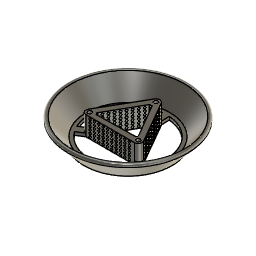
gaseta EMF medio v7 (Autodesk Fusion 360 design; units mm, degrees)
Autodesk Fusion 360 part; units mm, degrees
sketch "Boceto1" plane through (0, 0, 0) normal (0, 0, 1) x (1, 0, 0)
  circle A0 centre (0, 0) radius 55
  circle A1 centre (0, 35) radius 2
  circle A2 centre (-30.3109, -17.5) radius 2
  circle A3 centre (30.3109, -17.5) radius 2
  dimension "d1" = 110
  dimension "d2" = 4
  dimension "d4" = 360
  constraint coincident A0.centre origin
  measures "d1" diameter of A0
  measures "d2" diameter of A1
extrude "Extruir1" add sketch "Boceto1" along normal blind 4
sketch "Boceto2" plane through (0, 0, 0) normal (0, 1, 0) x (1, 0, 0)
  line L0 (55, 0) -> (78.3935, 0) construction
  line L1 (-55, 0) -> (55, 0) construction
  line L2 (55, 0) -> (74.2836, -22.9813)
  line L3 (70.7419, -25.9532) -> (51.4583, -2.9719)
  line L4 (51.4583, -2.9719) -> (55, 0)
  line L5 (-55, -4) -> (55, -4) construction
  arc A0 (70.7419, -25.9532) -> (74.2836, -22.9813) centre (72.5128, -24.4673) ccw
  dimension "d10" = 55
  dimension "d14" = 50
  dimension "d16" = 4
  constraint horizontal L0
  constraint parallel L2 L3
  measures "d10" distance of origin L0.start
  measures "d14" angle of L0 L2
  measures "d16" distance of L0 L5
revolve "Revolución1" add sketch "Boceto2" angle 360 about axis through (0, 0, 1.75) along (0, 0, 1)
sketch "Boceto3" plane through (0, 0, 4) normal (0, 0, 1) x (-1, 0, 0)
  circle A0 centre (0, 0) radius 52.321
  circle A1 centre (30.3109, 17.5) radius 2.5
  circle A2 centre (-30.3109, 17.5) radius 2.5
  line L0 (4.4101, -37.356) -> (34.7606, 15.2015)
  arc A3 (34.7534, 15.2057) -> (30.1462, 22.4973) centre (30.3109, 17.5) ccw
  line L1 (34.7606, 15.2015) -> (34.7534, 15.2057)
  line L2 (-0.0023, -25.0055) -> (21.6565, 12.5008)
  line L3 (21.6565, 12.5008) -> (-21.6543, 12.5047)
  arc A4 (34.7534, 15.2057) -> (30.1462, 22.4973) centre (30.3109, 17.5) ccw
  line L4 (30.1462, 22.4973) -> (-30.5452, 22.4945)
  arc A5 (-30.5452, 22.4945) -> (-34.6389, 15.0017) centre (-30.3098, 17.5012) ccw
  line L5 (-21.6543, 12.5047) -> (-0.0023, -25.0055)
  line L6 (-34.6389, 15.0017) -> (-4.2082, -37.7002)
  arc A6 (-4.2082, -37.7002) -> (4.4101, -37.356) centre (0, -35) ccw
  circle A7 centre (0, -35) radius 2.5
  dimension "d66" = 5
  dimension "d67" = 5
  dimension "d68" = 5
  constraint coincident L0 A6.end
  constraint coincident L6 A5.end
  constraint coincident L4.end A5.start
  constraint coincident A3.end A4.end
  constraint coincident L6.end A6.start
  constraint coincident A5.end L6.start
  constraint coincident L0.start A6.end
  constraint concentric A6 A7
  measures "d66" diameter of A1
  measures "d67" diameter of A2
  measures "d68" diameter of A7
extrude "Extruir2" add sketch "Boceto3" along normal blind 20 contours L0 A3 L1 A4 L4 A5 L6 A6 | L2 L3 L5
extrude "Extruir3" add sketch "Boceto3" along normal blind 20 contours L0 A3 L1 A4 L4 A5 L6 A6
extrude "Extruir4" cut sketch "Boceto3" against normal blind 30 contours A1 | A2 | A7
sketch "Boceto5" plane through (0, 0, 0) normal (0, 0, -1) x (1, 0, 0)
  circle A0 centre (-30.3109, 17.5) radius 2.5
  circle A1 centre (30.3109, 17.5) radius 2.5
  circle A2 centre (0, 0) radius 55
  line L0 (0.2076, -31) -> (27.1755, 15.0161)
  line L1 (27.1755, 15.0161) -> (-26.6179, 15.9631)
  line L2 (-26.6179, 15.9631) -> (0.2076, -31)
  arc A3 (-30.1462, 22.4973) -> (-34.7534, 15.2057) centre (-30.3109, 17.5) ccw
  line L3 (4.2082, -37.7002) -> (3.803, -47.8491)
  line L4 (-4.8254, -47.7568) -> (-4.4101, -37.356)
  line L5 (30.5452, 22.4945) -> (39.537, 27.218)
  line L6 (43.7713, 19.6995) -> (34.5563, 14.8588)
  line L7 (-34.7534, 15.2057) -> (-43.34, 20.6311)
  line L8 (-38.9459, 28.0573) -> (-30.1462, 22.4973)
  arc A4 (39.537, 27.218) -> (-38.9459, 28.0573) centre (0, 0) ccw
  arc A5 (-43.34, 20.6311) -> (-4.8254, -47.7568) centre (0, 0) ccw
  arc A6 (3.803, -47.8491) -> (43.7713, 19.6995) centre (0, 0) ccw
  line L9 (34.5563, 14.8588) -> (4.2082, -37.7002)
  line L10 (-4.4101, -37.356) -> (-34.7534, 15.2057)
  line L11 (-30.1462, 22.4973) -> (30.5452, 22.4945)
  circle A7 centre (0, -35) radius 2.5
  point P0 (0, -35)
  point P1 (30.3098, 17.5012)
  dimension "d31" = 4
  dimension "d32" = 4
  dimension "d33" = 4
  dimension "d34" = 96
  constraint coincident A3.end L7.start
  constraint coincident A3.start L8.end
  constraint coincident L5.end A5
  constraint concentric A4 A5
  constraint coincident L3.end A5
  constraint concentric A5 A6
  measures "d31" vertical distance of L0.start P0
  measures "d32" distance of L0.end P1
  measures "d33" distance of L1.end A0.centre
  measures "d34" diameter of A5
extrude "Extruir5" cut sketch "Boceto5" against normal blind 80 contours L0 L1 L2 | L3 L6 A6 L9 | L4 L7 A5 L10 | L5 L8 A4 L11
fillet "Empalme1" radius 2 3 edges at (27.1755, -15.0161, 12) (-26.6179, -15.9631, 12) (0.2076, 31, 12)
sketch "Boceto6" plane through (-19.4825, 11.2471, 0) normal (-0.866048, 0.49996, 0) x (-0.49996, -0.866048, 0)
  line L0 (30.5442, 24) -> (-30.1473, 24)
  line L1 (-30.1473, 24) -> (-30.1473, 4)
  line L2 (-30.1473, 4) -> (-30.1473, 0)
  line L3 (-30.1473, 0) -> (30.5442, 0)
  line L4 (30.5442, 0) -> (30.5442, 4)
  line L5 (30.5442, 4) -> (30.5442, 24)
  circle A0 centre (-25, 21.5) radius 1.35
  circle A1 centre (-19.4444, 21.5) radius 1.35
  circle A2 centre (-13.8889, 21.5) radius 1.35
  circle A3 centre (-8.3333, 21.5) radius 1.35
  circle A4 centre (-2.7778, 21.5) radius 1.35
  circle A5 centre (2.7778, 21.5) radius 1.35
  circle A6 centre (8.3333, 21.5) radius 1.35
  circle A7 centre (13.8889, 21.5) radius 1.35
  circle A8 centre (19.4444, 21.5) radius 1.35
  circle A9 centre (25, 21.5) radius 1.35
  circle A10 centre (-25, 17.7) radius 1.35
  circle A11 centre (-19.4444, 17.7) radius 1.35
  circle A12 centre (-13.8889, 17.7) radius 1.35
  circle A13 centre (-8.3333, 17.7) radius 1.35
  circle A14 centre (-2.7778, 17.7) radius 1.35
  circle A15 centre (2.7778, 17.7) radius 1.35
  circle A16 centre (8.3333, 17.7) radius 1.35
  circle A17 centre (13.8889, 17.7) radius 1.35
  circle A18 centre (19.4444, 17.7) radius 1.35
  circle A19 centre (25, 17.7) radius 1.35
  circle A20 centre (-25, 13.9) radius 1.35
  circle A21 centre (-19.4444, 13.9) radius 1.35
  circle A22 centre (-13.8889, 13.9) radius 1.35
  circle A23 centre (-8.3333, 13.9) radius 1.35
  circle A24 centre (-2.7778, 13.9) radius 1.35
  circle A25 centre (2.7778, 13.9) radius 1.35
  circle A26 centre (8.3333, 13.9) radius 1.35
  circle A27 centre (13.8889, 13.9) radius 1.35
  circle A28 centre (19.4444, 13.9) radius 1.35
  circle A29 centre (25, 13.9) radius 1.35
  circle A30 centre (-25, 10.1) radius 1.35
  circle A31 centre (-19.4444, 10.1) radius 1.35
  circle A32 centre (-13.8889, 10.1) radius 1.35
  circle A33 centre (-8.3333, 10.1) radius 1.35
  circle A34 centre (-2.7778, 10.1) radius 1.35
  circle A35 centre (2.7778, 10.1) radius 1.35
  circle A36 centre (8.3333, 10.1) radius 1.35
  circle A37 centre (13.8889, 10.1) radius 1.35
  circle A38 centre (19.4444, 10.1) radius 1.35
  circle A39 centre (25, 10.1) radius 1.35
  circle A40 centre (-25, 6.3) radius 1.35
  circle A41 centre (-19.4444, 6.3) radius 1.35
  circle A42 centre (-13.8889, 6.3) radius 1.35
  circle A43 centre (-8.3333, 6.3) radius 1.35
  circle A44 centre (-2.7778, 6.3) radius 1.35
  circle A45 centre (2.7778, 6.3) radius 1.35
  circle A46 centre (8.3333, 6.3) radius 1.35
  circle A47 centre (13.8889, 6.3) radius 1.35
  circle A48 centre (19.4444, 6.3) radius 1.35
  circle A49 centre (25, 6.3) radius 1.35
  circle A50 centre (-25, 2.5) radius 1.35
  circle A51 centre (-19.4444, 2.5) radius 1.35
  circle A52 centre (-13.8889, 2.5) radius 1.35
  circle A53 centre (-8.3333, 2.5) radius 1.35
  circle A54 centre (-2.7778, 2.5) radius 1.35
  circle A55 centre (2.7778, 2.5) radius 1.35
  circle A56 centre (8.3333, 2.5) radius 1.35
  circle A57 centre (13.8889, 2.5) radius 1.35
  circle A58 centre (19.4444, 2.5) radius 1.35
  circle A59 centre (25, 2.5) radius 1.35
  dimension "d39" = 2.7
  dimension "d42" = 50
  dimension "d43" = -19
  dimension "d44" = 21.5
  dimension "d45" = 25
  measures "d39" diameter of A0
  measures "d44" vertical distance of origin A0.centre
  measures "d45" horizontal distance of origin A0.centre
extrude "Extruir6" cut sketch "Boceto6" against normal blind 9 contours A0 | A1 | A2 | A3 | A4 | A5 | A6 | A7 | A8 | A9 | A10 | A11 | A12 | A13 | A14 | A15 | A16 | A17 | A18 | A19 | A20 | A21 | A22 | A23 | A24 | A25 | A26 | A27 | A28 | A29 | A30 | A31 | A32 | A33 | A34 | A35 | A36 | A37 | A38 | A39 | A40 | A41 | A42 | A43 | A44 | A45 | A46 | A47 | A48 | A49 | A50 | A51 | A52 | A53 | A54 | A55 | A56 | A57 | A58 | A59
sketch "Boceto7" plane through (0.001, -22.4959, 0) normal (0.000046, -1, 0) x (1, 0.000046, 0)
  line L0 (30.5441, 4) -> (30.5441, 24)
  line L1 (30.5441, 24) -> (-30.1473, 24)
  line L2 (-30.1473, 24) -> (-30.1473, 4)
  line L3 (-30.1473, 4) -> (-30.1473, 0)
  line L4 (-30.1473, 0) -> (30.5442, 0)
  line L5 (30.5442, 0) -> (30.5441, 4)
  circle A0 centre (-25, 21.5) radius 1.35
  circle A1 centre (-19.5556, 21.5) radius 1.35
  circle A2 centre (-14.1111, 21.5) radius 1.35
  circle A3 centre (-8.6667, 21.5) radius 1.35
  circle A4 centre (-3.2222, 21.5) radius 1.35
  circle A5 centre (2.2222, 21.5) radius 1.35
  circle A6 centre (7.6667, 21.5) radius 1.35
  circle A7 centre (13.1111, 21.5) radius 1.35
  circle A8 centre (18.5556, 21.5) radius 1.35
  circle A9 centre (24, 21.5) radius 1.35
  circle A10 centre (-25, 17.7) radius 1.35
  circle A11 centre (-19.5556, 17.7) radius 1.35
  circle A12 centre (-14.1111, 17.7) radius 1.35
  circle A13 centre (-8.6667, 17.7) radius 1.35
  circle A14 centre (-3.2222, 17.7) radius 1.35
  circle A15 centre (2.2222, 17.7) radius 1.35
  circle A16 centre (7.6667, 17.7) radius 1.35
  circle A17 centre (13.1111, 17.7) radius 1.35
  circle A18 centre (18.5556, 17.7) radius 1.35
  circle A19 centre (24, 17.7) radius 1.35
  circle A20 centre (-25, 13.9) radius 1.35
  circle A21 centre (-19.5556, 13.9) radius 1.35
  circle A22 centre (-14.1111, 13.9) radius 1.35
  circle A23 centre (-8.6667, 13.9) radius 1.35
  circle A24 centre (-3.2222, 13.9) radius 1.35
  circle A25 centre (2.2222, 13.9) radius 1.35
  circle A26 centre (7.6667, 13.9) radius 1.35
  circle A27 centre (13.1111, 13.9) radius 1.35
  circle A28 centre (18.5556, 13.9) radius 1.35
  circle A29 centre (24, 13.9) radius 1.35
  circle A30 centre (-25, 10.1) radius 1.35
  circle A31 centre (-19.5556, 10.1) radius 1.35
  circle A32 centre (-14.1111, 10.1) radius 1.35
  circle A33 centre (-8.6667, 10.1) radius 1.35
  circle A34 centre (-3.2222, 10.1) radius 1.35
  circle A35 centre (2.2222, 10.1) radius 1.35
  circle A36 centre (7.6667, 10.1) radius 1.35
  circle A37 centre (13.1111, 10.1) radius 1.35
  circle A38 centre (18.5556, 10.1) radius 1.35
  circle A39 centre (24, 10.1) radius 1.35
  circle A40 centre (-25, 6.3) radius 1.35
  circle A41 centre (-19.5556, 6.3) radius 1.35
  circle A42 centre (-14.1111, 6.3) radius 1.35
  circle A43 centre (-8.6667, 6.3) radius 1.35
  circle A44 centre (-3.2222, 6.3) radius 1.35
  circle A45 centre (2.2222, 6.3) radius 1.35
  circle A46 centre (7.6667, 6.3) radius 1.35
  circle A47 centre (13.1111, 6.3) radius 1.35
  circle A48 centre (18.5556, 6.3) radius 1.35
  circle A49 centre (24, 6.3) radius 1.35
  circle A50 centre (-25, 2.5) radius 1.35
  circle A51 centre (-19.5556, 2.5) radius 1.35
  circle A52 centre (-14.1111, 2.5) radius 1.35
  circle A53 centre (-8.6667, 2.5) radius 1.35
  circle A54 centre (-3.2222, 2.5) radius 1.35
  circle A55 centre (2.2222, 2.5) radius 1.35
  circle A56 centre (7.6667, 2.5) radius 1.35
  circle A57 centre (13.1111, 2.5) radius 1.35
  circle A58 centre (18.5556, 2.5) radius 1.35
  circle A59 centre (24, 2.5) radius 1.35
  dimension "d48" = 2.7
  dimension "d49" = 25
  dimension "d50" = 21.5
  dimension "d53" = 49
  dimension "d54" = -19
  measures "d48" diameter of A0
  measures "d49" horizontal distance of origin A0.centre
  measures "d50" vertical distance of origin A0.centre
extrude "Extruir7" cut sketch "Boceto7" against normal blind 9 contours A0 | A1 | A2 | A3 | A4 | A5 | A6 | A7 | A8 | A9 | A10 | A11 | A12 | A13 | A14 | A15 | A16 | A17 | A18 | A19 | A20 | A21 | A22 | A23 | A24 | A25 | A26 | A27 | A28 | A29 | A30 | A31 | A32 | A33 | A34 | A35 | A36 | A37 | A38 | A39 | A40 | A41 | A42 | A43 | A44 | A45 | A46 | A47 | A48 | A49 | A50 | A51 | A52 | A53 | A54 | A55 | A56 | A57 | A58 | A59
sketch "Boceto8" plane through (19.4815, 11.2488, 0) normal (0.866002, 0.50004, 0) x (-0.50004, 0.866002, 0)
  line L0 (30.5442, 24) -> (-30.3124, 24)
  line L1 (-30.3124, 24) -> (-30.3124, 4)
  line L2 (-30.3124, 4) -> (-30.1473, 4)
  line L3 (-30.1473, 4) -> (-30.1473, 0)
  line L4 (-30.1473, 0) -> (30.5442, 0)
  line L5 (30.5442, 0) -> (30.5442, 4)
  line L6 (30.5442, 4) -> (30.5442, 24)
  circle A0 centre (-25, 21.5) radius 1.35
  circle A1 centre (-19.5556, 21.5) radius 1.35
  circle A2 centre (-14.1111, 21.5) radius 1.35
  circle A3 centre (-8.6667, 21.5) radius 1.35
  circle A4 centre (-3.2222, 21.5) radius 1.35
  circle A5 centre (2.2222, 21.5) radius 1.35
  circle A6 centre (7.6667, 21.5) radius 1.35
  circle A7 centre (13.1111, 21.5) radius 1.35
  circle A8 centre (18.5556, 21.5) radius 1.35
  circle A9 centre (24, 21.5) radius 1.35
  circle A10 centre (-25, 17.7) radius 1.35
  circle A11 centre (-19.5556, 17.7) radius 1.35
  circle A12 centre (-14.1111, 17.7) radius 1.35
  circle A13 centre (-8.6667, 17.7) radius 1.35
  circle A14 centre (-3.2222, 17.7) radius 1.35
  circle A15 centre (2.2222, 17.7) radius 1.35
  circle A16 centre (7.6667, 17.7) radius 1.35
  circle A17 centre (13.1111, 17.7) radius 1.35
  circle A18 centre (18.5556, 17.7) radius 1.35
  circle A19 centre (24, 17.7) radius 1.35
  circle A20 centre (-25, 13.9) radius 1.35
  circle A21 centre (-19.5556, 13.9) radius 1.35
  circle A22 centre (-14.1111, 13.9) radius 1.35
  circle A23 centre (-8.6667, 13.9) radius 1.35
  circle A24 centre (-3.2222, 13.9) radius 1.35
  circle A25 centre (2.2222, 13.9) radius 1.35
  circle A26 centre (7.6667, 13.9) radius 1.35
  circle A27 centre (13.1111, 13.9) radius 1.35
  circle A28 centre (18.5556, 13.9) radius 1.35
  circle A29 centre (24, 13.9) radius 1.35
  circle A30 centre (-25, 10.1) radius 1.35
  circle A31 centre (-19.5556, 10.1) radius 1.35
  circle A32 centre (-14.1111, 10.1) radius 1.35
  circle A33 centre (-8.6667, 10.1) radius 1.35
  circle A34 centre (-3.2222, 10.1) radius 1.35
  circle A35 centre (2.2222, 10.1) radius 1.35
  circle A36 centre (7.6667, 10.1) radius 1.35
  circle A37 centre (13.1111, 10.1) radius 1.35
  circle A38 centre (18.5556, 10.1) radius 1.35
  circle A39 centre (24, 10.1) radius 1.35
  circle A40 centre (-25, 6.3) radius 1.35
  circle A41 centre (-19.5556, 6.3) radius 1.35
  circle A42 centre (-14.1111, 6.3) radius 1.35
  circle A43 centre (-8.6667, 6.3) radius 1.35
  circle A44 centre (-3.2222, 6.3) radius 1.35
  circle A45 centre (2.2222, 6.3) radius 1.35
  circle A46 centre (7.6667, 6.3) radius 1.35
  circle A47 centre (13.1111, 6.3) radius 1.35
  circle A48 centre (18.5556, 6.3) radius 1.35
  circle A49 centre (24, 6.3) radius 1.35
  circle A50 centre (-25, 2.5) radius 1.35
  circle A51 centre (-19.5556, 2.5) radius 1.35
  circle A52 centre (-14.1111, 2.5) radius 1.35
  circle A53 centre (-8.6667, 2.5) radius 1.35
  circle A54 centre (-3.2222, 2.5) radius 1.35
  circle A55 centre (2.2222, 2.5) radius 1.35
  circle A56 centre (7.6667, 2.5) radius 1.35
  circle A57 centre (13.1111, 2.5) radius 1.35
  circle A58 centre (18.5556, 2.5) radius 1.35
  circle A59 centre (24, 2.5) radius 1.35
  dimension "d57" = 2.7
  dimension "d58" = 21.5
  dimension "d59" = 25
  dimension "d62" = 49
  dimension "d63" = -19
  measures "d57" diameter of A0
  measures "d58" vertical distance of origin A0.centre
  measures "d59" horizontal distance of origin A0.centre
extrude "Extruir8" cut sketch "Boceto8" against normal blind 9 contours A0 | A1 | A2 | A3 | A4 | A5 | A6 | A7 | A8 | A9 | A10 | A11 | A12 | A13 | A14 | A15 | A16 | A17 | A18 | A19 | A20 | A21 | A22 | A23 | A24 | A25 | A26 | A27 | A28 | A29 | A30 | A31 | A32 | A33 | A34 | A35 | A36 | A37 | A38 | A39 | A40 | A41 | A42 | A43 | A44 | A45 | A46 | A47 | A48 | A49 | A50 | A51 | A52 | A53 | A54 | A55 | A56 | A57 | A58 | A59
